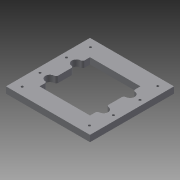
# Autodesk Inventor part: core xy carriage
Saved by Autodesk Inventor 2014 SP1 (Build 180222100, 222)
## iProperties
Created: 2014-09-21
Part Number: core xy carriage
Material: Generic
Document SubType Name: Modeling
Designer: Mon
Density: 1 g/cm^3
Appearance: Default
Author: Mon
Autodesk Inventor part; units mm, degrees
ref_plane "YZ Plane" through (0, 0, 0) normal (1, 0, 0) x (0, 1, 0)
ref_plane "XZ Plane" through (0, 0, 0) normal (0, 1, 0) x (-1, 0, 0)
ref_plane "XY Plane" through (0, 0, 0) normal (0, 0, 1) x (1, 0, 0)
sketch "Sketch1" plane through (0, 0, 0) normal (0, 1, 0) x (-1, 0, 0)
  line L0 (50.7798, 12.6798) -> (12.6798, 12.6798)
  line L1 (50.7798, 16.7388) -> (50.7798, 12.6798)
  arc A0 (52.1898, 18.2361) -> (50.7798, 16.7388) centre (52.2798, 16.7388) ccw
  arc A1 (52.1898, 18.2361) -> (52.1898, 25.2235) centre (51.9798, 21.7298) ccw
  arc A2 (50.7798, 26.7208) -> (52.1898, 25.2235) centre (52.2798, 26.7208) ccw
  arc A3 (52.1898, 38.2361) -> (50.7798, 36.7388) centre (52.2798, 36.7388) ccw
  arc A4 (52.1898, 38.2361) -> (52.1898, 45.2235) centre (51.9798, 41.7298) ccw
  arc A5 (50.7798, 46.7208) -> (52.1898, 45.2235) centre (52.2798, 46.7208) ccw
  line L2 (12.6798, 50.7798) -> (50.7798, 50.7798)
  line L3 (12.6798, 46.7208) -> (12.6798, 50.7798)
  arc A6 (11.2698, 45.2235) -> (12.6798, 46.7208) centre (11.1798, 46.7208) ccw
  arc A7 (11.2698, 45.2235) -> (11.2698, 38.2361) centre (11.4798, 41.7298) ccw
  arc A8 (12.6798, 36.7388) -> (11.2698, 38.2361) centre (11.1798, 36.7388) ccw
  arc A9 (11.2698, 25.2235) -> (12.6798, 26.7208) centre (11.1798, 26.7208) ccw
  arc A10 (11.2698, 25.2235) -> (11.2698, 18.2361) centre (11.4798, 21.7298) ccw
  arc A11 (12.6798, 16.7388) -> (11.2698, 18.2361) centre (11.1798, 16.7388) ccw
  line L4 (-0.0202, 63.4798) -> (63.4798, 63.4798)
  line L5 (63.4798, 63.4798) -> (63.4798, -0.0202)
  line L6 (63.4798, -0.0202) -> (-0.0202, -0.0202)
  line L7 (-0.0202, -0.0202) -> (-0.0202, 63.4798)
  circle A12 centre (6.3298, 5.9173) radius 0.875
  circle A13 centre (57.1298, 5.9173) radius 0.875
  circle A14 centre (57.1298, 57.5423) radius 0.875
  circle A15 centre (6.3298, 57.5423) radius 0.875
  circle A16 centre (3.9798, 41.7298) radius 0.875
  circle A17 centre (59.4798, 41.7298) radius 0.875
  circle A18 centre (59.4798, 21.7298) radius 0.875
  circle A19 centre (3.9798, 21.7298) radius 0.875
  line L8 (12.6798, 12.6798) -> (12.6798, 16.7388)
  line L9 (12.6798, 26.7208) -> (12.6798, 36.7388)
  line L10 (50.7798, 50.7798) -> (50.7798, 46.7208)
  line L11 (50.7798, 36.7388) -> (50.7798, 26.7208)
  point P0 (0, 0)
  constraints: 24 end point, 24 point on circle, 20 centre point
extrude "Extrusion1" add sketch "Sketch1" along normal blind 4.7625
body "Solid1"
